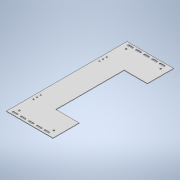
# Autodesk Inventor part: lid
Saved by Autodesk Inventor 2020 (Build 240168000, 168)
## iProperties
Created: 2021-11-11
Part Number: lid
Material: Generic
Document SubType Name: Modeling
Designer: 17185
Density: 1 g/cm^3
Appearance: Default
Author: 17185
Autodesk Inventor part; units mm, degrees
ref_plane "YZ Plane" through (0, 0, 0) normal (1, 0, 0) x (0, 1, 0)
ref_plane "XZ Plane" through (0, 0, 0) normal (0, 1, 0) x (-1, 0, 0)
ref_plane "XY Plane" through (0, 0, 0) normal (0, 0, 1) x (1, 0, 0)
sketch "Sketch1" plane through (0, 0, 0) normal (0, 1, 0) x (-1, 0, 0)
  line L0 (147.066, 381) -> (0, 381)
  line L1 (-147.066, 33.688) -> (-147.066, -381)
  line L2 (-147.066, -381) -> (147.066, -381)
  line L3 (147.066, -381) -> (147.066, 381)
  line L4 (147.066, 381) -> (-147.066, -381) construction
  line L5 (136.271, -185.928) -> (115.951, -185.928) construction
  line L6 (115.951, -185.928) -> (115.951, -231.648) construction
  line L7 (115.951, -231.648) -> (136.271, -231.648) construction
  line L8 (136.271, -231.648) -> (136.271, -185.928) construction
  line L9 (136.271, -185.928) -> (115.951, -231.648) construction
  line L10 (115.951, -185.928) -> (136.271, -231.648) construction
  circle A0 centre (126.111, -231.648) radius 3.556
  circle A1 centre (126.111, -185.928) radius 3.556
  circle A2 centre (126.111, -208.788) radius 3.556
  line L11 (0, 0) -> (147.066, 0) construction
  line L12 (136.271, 231.648) -> (115.951, 231.648) construction
  line L13 (115.951, 231.648) -> (115.951, 185.928) construction
  line L14 (115.951, 185.928) -> (136.271, 185.928) construction
  line L15 (136.271, 185.928) -> (136.271, 231.648) construction
  line L16 (136.271, 231.648) -> (115.951, 185.928) construction
  line L17 (115.951, 231.648) -> (136.271, 185.928) construction
  circle A3 centre (126.111, 231.648) radius 3.556
  circle A4 centre (126.111, 208.788) radius 3.556
  circle A5 centre (126.111, 185.928) radius 3.556
  line L18 (0, 381) -> (-147.066, 381)
  line L19 (-147.066, 381) -> (-147.066, 33.688)
  line L20 (0, 215.9) -> (-147.066, 215.9)
  line L21 (-147.066, 215.9) -> (-147.066, -215.9)
  line L22 (-147.066, -215.9) -> (0, -215.9)
  line L23 (0, -215.9) -> (0, 215.9)
  line L24 (0, 215.9) -> (-147.066, -215.9) construction
  line L25 (-147.066, 215.9) -> (0, -215.9) construction
  point P0 (-73.533, 0)
  dimension "d1" = 294.132
  dimension "d8" = 20.955
  dimension "d9" = 762
  dimension "d10" = 20.32
  dimension "d11" = 45.72
  dimension "d12" = 7.112
  dimension "d13" = 7.112
  dimension "d14" = 7.112
  dimension "d15" = 149.352
  dimension "d16" = 45.72
  dimension "d17" = 149.352
  dimension "d18" = 7.112
  dimension "d19" = 7.112
  dimension "d20" = 7.112
  dimension "d21" = 431.8
  dimension "d22" = 147.066
  dimension "d23" = 0
  constraints: 52 end point, 13 midpoint, 8 parallel, 6 centre point, 5 perpendicular, 4 horizontal, 2 coincident, 1 point on line
  measures "d1" distance of L1.end L2.end
  measures "d8" distance from line of L3 point (126.111, -208.788)
  measures "d9" distance between parallel lines of L0 L2
  measures "d10" distance of L6.end L7.end
  measures "d11" distance of L5.end L6.end
  measures "d12" diameter of A0
  measures "d13" diameter of A1
  measures "d14" diameter of A2
  measures "d15" distance from line of A0.centre L2
  measures "d16" distance of L12.end L13.end
  measures "d17" distance between parallel lines of L12 L0
  measures "d18" diameter of A3
  measures "d19" diameter of A4
  measures "d20" diameter of A5
  measures "d21" distance of L22.end L20.start
  measures "d22" distance of L21.end L22.end
  measures "d23" vertical distance of L11.start point (-73.533, 0)
extrude "Extrusion1" add sketch "Sketch1" along normal blind 3.175 contours L3 L2 L1 L22 L23 L20 L19 L18 L0
sketch "Sketch2" plane through (0, 3.175, 0) normal (0, 1, 0) x (1, 0, 0)
  line L0 (-121.666, 364.3122) -> (-96.266, 364.3122) construction
  line L1 (-121.666, 359.8672) -> (-96.266, 359.8672)
  line L2 (-96.266, 368.7572) -> (-121.666, 368.7572)
  arc A0 (-121.666, 368.7572) -> (-121.666, 359.8672) centre (-121.666, 364.3122) ccw
  arc A1 (-96.266, 359.8672) -> (-96.266, 368.7572) centre (-96.266, 364.3122) ccw
  line L3 (147.066, 381) -> (-147.066, 381) projected
  line L4 (-70.866, 364.3122) -> (-45.466, 364.3122) construction
  line L5 (-70.866, 359.8672) -> (-45.466, 359.8672)
  line L6 (-45.466, 368.7572) -> (-70.866, 368.7572)
  arc A2 (-70.866, 368.7572) -> (-70.866, 359.8672) centre (-70.866, 364.3122) ccw
  arc A3 (-45.466, 359.8672) -> (-45.466, 368.7572) centre (-45.466, 364.3122) ccw
  line L7 (-20.066, 364.3122) -> (5.334, 364.3122) construction
  line L8 (-20.066, 359.8672) -> (5.334, 359.8672)
  line L9 (5.334, 368.7572) -> (-20.066, 368.7572)
  arc A4 (-20.066, 368.7572) -> (-20.066, 359.8672) centre (-20.066, 364.3122) ccw
  arc A5 (5.334, 359.8672) -> (5.334, 368.7572) centre (5.334, 364.3122) ccw
  line L10 (30.734, 364.3122) -> (56.134, 364.3122) construction
  line L11 (30.734, 359.8672) -> (56.134, 359.8672)
  line L12 (56.134, 368.7572) -> (30.734, 368.7572)
  arc A6 (30.734, 368.7572) -> (30.734, 359.8672) centre (30.734, 364.3122) ccw
  arc A7 (56.134, 359.8672) -> (56.134, 368.7572) centre (56.134, 364.3122) ccw
  line L13 (-147.066, 381) -> (-147.066, -381) projected
  line L14 (0, 0) -> (-147.066, 0) construction
  line L15 (-121.666, -364.3122) -> (-96.266, -364.3122) construction
  line L16 (-121.666, -359.8672) -> (-96.266, -359.8672)
  line L17 (-96.266, -368.7572) -> (-121.666, -368.7572)
  arc A8 (-121.666, -359.8672) -> (-121.666, -368.7572) centre (-121.666, -364.3122) ccw
  arc A9 (-96.266, -368.7572) -> (-96.266, -359.8672) centre (-96.266, -364.3122) ccw
  line L18 (-70.866, -364.3122) -> (-45.466, -364.3122) construction
  line L19 (-70.866, -359.8672) -> (-45.466, -359.8672)
  line L20 (-45.466, -368.7572) -> (-70.866, -368.7572)
  arc A10 (-70.866, -359.8672) -> (-70.866, -368.7572) centre (-70.866, -364.3122) ccw
  arc A11 (-45.466, -368.7572) -> (-45.466, -359.8672) centre (-45.466, -364.3122) ccw
  line L21 (-20.066, -364.3122) -> (5.334, -364.3122) construction
  line L22 (-20.066, -359.8672) -> (5.334, -359.8672)
  line L23 (5.334, -368.7572) -> (-20.066, -368.7572)
  arc A12 (-20.066, -359.8672) -> (-20.066, -368.7572) centre (-20.066, -364.3122) ccw
  arc A13 (5.334, -368.7572) -> (5.334, -359.8672) centre (5.334, -364.3122) ccw
  line L24 (30.734, -364.3122) -> (56.134, -364.3122) construction
  line L25 (30.734, -359.8672) -> (56.134, -359.8672)
  line L26 (56.134, -368.7572) -> (30.734, -368.7572)
  arc A14 (30.734, -359.8672) -> (30.734, -368.7572) centre (30.734, -364.3122) ccw
  arc A15 (56.134, -368.7572) -> (56.134, -359.8672) centre (56.134, -364.3122) ccw
  circle A16 centre (-108.966, 337.185) radius 4.7625
  circle A17 centre (108.966, 337.185) radius 4.7625
  line L27 (147.066, 215.9) -> (147.066, 381) projected
  circle A18 centre (-108.966, -337.185) radius 4.7625
  circle A19 centre (108.966, -337.185) radius 4.7625
  line L28 (78.7859, 364.3122) -> (104.1859, 364.3122) construction
  line L29 (78.7859, 359.8672) -> (104.1859, 359.8672)
  line L30 (104.1859, 368.7572) -> (78.7859, 368.7572)
  arc A20 (78.7859, 368.7572) -> (78.7859, 359.8672) centre (78.7859, 364.3122) ccw
  arc A21 (104.1859, 359.8672) -> (104.1859, 368.7572) centre (104.1859, 364.3122) ccw
  line L31 (78.7859, -364.3122) -> (104.1859, -364.3122) construction
  line L32 (78.7859, -359.8672) -> (104.1859, -359.8672)
  line L33 (104.1859, -368.7572) -> (78.7859, -368.7572)
  arc A22 (78.7859, -359.8672) -> (78.7859, -368.7572) centre (78.7859, -364.3122) ccw
  arc A23 (104.1859, -368.7572) -> (104.1859, -359.8672) centre (104.1859, -364.3122) ccw
  point P0 (-108.966, 364.3122)
  point P1 (-58.166, 364.3122)
  point P2 (-7.366, 364.3122)
  point P3 (43.434, 364.3122)
  point P4 (-108.966, -364.3122)
  point P5 (-58.166, -364.3122)
  point P6 (-7.366, -364.3122)
  point P7 (43.434, -364.3122)
  point P8 (91.4859, 364.3122)
  point P9 (91.4859, -364.3122)
  dimension "d24" = 8.89
  dimension "d25" = 16.6878
  dimension "d26" = 25.4
  dimension "d27" = 25.4
  dimension "d28" = 8.89
  dimension "d29" = 25.4
  dimension "d30" = 8.89
  dimension "d31" = 25.4
  dimension "d32" = 8.89
  dimension "d33" = 25.4
  dimension "d34" = 25.4
  dimension "d35" = 25.4
  dimension "d36" = 25.4
  dimension "d42" = 9.525
  dimension "d43" = 43.815
  dimension "d44" = 38.1
  dimension "d45" = 9.525
  dimension "d46" = 43.815
  dimension "d47" = 38.1
  dimension "d48" = 25.4
  dimension "d49" = 4.445
  constraints: 82 end point, 40 point on circle, 37 symmetric about line, 24 centre point, 20 tangent, 8 point on line, 6 midpoint, 5 parallel, 3 horizontal, 12 other
  measures "d24" diameter of A1
  measures "d25" distance between parallel lines of L0 L3
  measures "d26" distance of L0.start L0.end
  measures "d27" distance of L4.start L4.end
  measures "d28" diameter of A3
  measures "d29" distance of L7.start L7.end
  measures "d30" diameter of A5
  measures "d31" distance of L10.start L10.end
  measures "d32" diameter of A7
  measures "d33" distance of L4.start L0.end
  measures "d34" distance of L7.start L4.end
  measures "d35" distance of L10.start L7.end
  measures "d36" distance from line of L13 L0.start
  measures "d42" diameter of A16
  measures "d43" distance from line of L3 A16.centre
  measures "d44" distance from line of A16.centre L13
  measures "d45" diameter of A17
  measures "d46" distance from line of L3 A17.centre
  measures "d47" distance from line of A17.centre L27
  measures "d48" distance of L28.start L28.end
  measures "d49" radius of A20
extrude "Extrusion2" cut sketch "Sketch2" against normal blind 3.175
equation "\"d12\" = d13"
equation "\"d14\" = d13"
equation "\"d16\" = d11"
equation "\"d17\" = d15"
equation "\"d18\" = d13"
equation "\"d19\" = d13"
equation "\"d20\" = d13"
equation "\"d27\" = d26"
equation "\"d29\" = d26"
equation "\"d31\" = d26"
equation "\"d33\" = d36"
equation "\"d34\" = d36"
equation "\"d35\" = d36"
equation "\"d45\" = d42"
equation "\"d46\" = d43"
equation "\"d47\" = d44"
equation "\"d48\" = d31"
equation "\"d49\" = 0.5 * d32"
body "Solid1"
